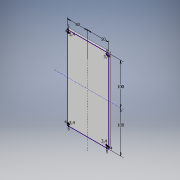
# Autodesk Inventor part: Chassis-2
Saved by Autodesk Inventor 2018 (Build 220112000, 112)
## iProperties
Created: 2018-01-20
Part Number: Chassis-2
Material: Generisch
Document SubType Name: Modeling
Designer: fhinstall
Density: 1 g/cm^3
Appearance: Vorgabe
Author: fhinstall
Autodesk Inventor part; units mm, degrees
ref_plane "YZ Plane" through (0, 0, 0) normal (1, 0, 0) x (0, 1, 0)
ref_plane "XZ Plane" through (0, 0, 0) normal (0, 1, 0) x (-1, 0, 0)
ref_plane "XY Plane" through (0, 0, 0) normal (0, 0, 1) x (1, 0, 0)
sketch "Skizze1" plane through (0, 0, 0) normal (0, 1, 0) x (-1, 0, 0)
  line L0 (50, 100) -> (50, -100)
  line L1 (50, -100) -> (-50, -100)
  line L2 (-50, -100) -> (-50, 100)
  line L3 (-50, 100) -> (50, 100)
  line L4 (0, 61.8387) -> (0, -129.7607) construction
  line L5 (83.0665, 0) -> (-88.5254, 0) construction
  circle A0 centre (46, 95) radius 1.7
  circle A1 centre (-46, 95) radius 1.7
  circle A2 centre (-46, -95) radius 1.7
  circle A3 centre (46, -95) radius 1.7
  point P0 (0, 0)
  dimension "d1" = 50
  dimension "d2" = 50
  dimension "d3" = 100
  dimension "d4" = 100
  dimension "d7" = 3.4
  dimension "d8" = 4
  dimension "d9" = 5
  dimension "d10" = 3.4
  dimension "d11" = 4
  dimension "d12" = 5
  dimension "d13" = 3.4
  dimension "d14" = 4
  dimension "d15" = 5
  dimension "d16" = 3.4
  dimension "d17" = 5
  dimension "d18" = 4
  constraints: 12 end point, 4 centre point, 2 perpendicular, 2 point on line, 2 vertical, 1 horizontal
  measures "d1" distance between parallel lines of L0 L4
  measures "d2" distance between parallel lines of L2 L4
  measures "d3" distance between parallel lines of L5 L3
  measures "d4" distance between parallel lines of L5 L1
  measures "d7" diameter of A0
  measures "d8" distance from line of L0 A0.centre
  measures "d9" distance from line of L3 A0.centre
  measures "d10" diameter of A1
  measures "d11" distance from line of L2 A1.centre
  measures "d12" distance from line of L3 A1.centre
  measures "d13" diameter of A2
  measures "d14" distance from line of L2 A2.centre
  measures "d15" distance from line of L1 A2.centre
  measures "d16" diameter of A3
  measures "d17" distance from line of L1 A3.centre
  measures "d18" distance from line of L0 A3.centre
extrude "Extrusion1" add sketch "Skizze1" along normal blind 5 contours L0 L1 L2 L3 | A0 | A1 | A2 | A3
extrude "Extrusion2" cut sketch "Skizze1" along normal blind 10 contours A0 | A1 | A2 | A3
